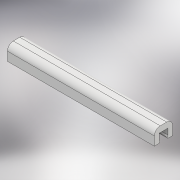
# Autodesk Inventor part: ForceStopper
Saved by Autodesk Inventor 2018.2 (Build 222227000, 227)
## iProperties
Created: 2018-04-02
Part Number: ForceStopper
Material: ABS Plastic
Document SubType Name: Modeling
Designer: Muchen He
Density: 1.06 g/cm^3
Appearance: Smooth - White
Author: Muchen He
Autodesk Inventor part; units mm, degrees
ref_plane "YZ Plane" through (0, 0, 0) normal (1, 0, 0) x (0, 1, 0)
ref_plane "XZ Plane" through (0, 0, 0) normal (0, 1, 0) x (-1, 0, 0)
ref_plane "XY Plane" through (0, 0, 0) normal (0, 0, 1) x (1, 0, 0)
sketch "Sketch1" plane through (0, 0, 0) normal (1, 0, 0) x (0, 1, 0)
  line L0 (1.5, -2) -> (-1.5, -2)
  line L1 (1.5, -2) -> (1.5, -4)
  line L2 (1.5, -4) -> (1.2, -4.5)
  line L3 (1.2, -4.5) -> (1.5, -5)
  line L4 (1.5, -5) -> (3.1, -5)
  line L5 (3.1, -5) -> (3.1, 0)
  line L6 (3.1, 0) -> (-3.1, 0)
  line L7 (-3.1, 0) -> (-3.1, -5)
  line L8 (-3.1, -5) -> (-1.5, -5)
  line L9 (-1.5, -5) -> (-1.2, -4.5)
  line L10 (-1.2, -4.5) -> (-1.5, -4)
  line L11 (-1.5, -4) -> (-1.5, -2)
  point P0 (0, 0)
  point P1 (0, -2)
  dimension "d0" = 3
  dimension "d1" = 2
  dimension "d2" = 1.6
  dimension "d3" = 1.6
  dimension "d4" = 0.3
  dimension "d5" = 3
  dimension "d6" = 2
  constraints: 24 end point, 4 perpendicular, 3 parallel, 3 point on line, 3 vertical alignment, 2 horizontal alignment, 2 midpoint, 1 horizontal, 1 vertical
  measures "d0" distance of L0.start L0.end
  measures "d1" distance between parallel lines of L0 L6
  measures "d2" distance between parallel lines of L11 L7
  measures "d3" distance between parallel lines of L5 L1
  measures "d4" horizontal distance of L8.end L9.end
  measures "d5" distance between parallel lines of L0 L8
  measures "d6" distance of L10.end L0.end
extrude "Extrusion1" add sketch "Sketch1" along normal blind 50
fillet "Fillet1" radius 2 2 edges at (25, 3.1, 0) (25, -3.1, 0)
body "Solid1"
